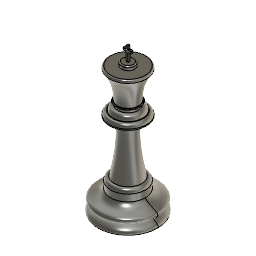
King (Autodesk Fusion 360 design; units mm, degrees)
part number: 2026-07-10-20-48-19-611
Autodesk Fusion 360 part; units mm, degrees
sketch "Pawn" plane through (0, 0, 0) normal (1, 0, 0) x (0, 1, 0)
  circle A0 through (0, 53, -10) (0, 61.6603, 5) (0, 44.3397, 5)
  line L0 (0, 43, 8.8) -> (0, 43, -8)
  line L1 (0, 40, -11) -> (0, 38.5991, -11)
  line L2 (0, 38.5991, -11) -> (0, 38.5991, 11.8)
  line L3 (0, 38.5991, 11.8) -> (0, 40, 11.8)
  arc A1 through (0, 43, 8.8) (0, 42.1213, 10.9213) (0, 40, 11.8)
  arc A2 through (0, 40, -11) (0, 42.1213, -10.1213) (0, 43, -8)
  arc A3 through (0, 13, 12) (0, 24.9602, 5.3081) (0, 38.5991, 3.9628)
  arc A4 through (0, 38.5991, -4.0372) (0, 24.9602, -5.3824) (0, 13, -12.0743)
  line L4 (0, 13, 14) -> (0, 13, -14)
  line L5 (0, 13, -14) -> (0, 9, -14)
  line L6 (0, 9, -14) -> (0, 9, 14)
  line L7 (0, 9, 14) -> (0, 13, 14)
  spline S0 degree 5 poles (0, 9, 14) (0, 8.9851, 14.1785) (0, 8.9515, 14.5305) (0, 8.8897, 15.0438) (0, 8.784, 15.698) (0, 8.6104, 16.4619) (0, 8.3911, 17.1666) (0, 8.1219, 17.8066) (0, 7.7992, 18.3771) (0, 7.4234, 18.8788) (0, 6.9978, 19.3158) (0, 6.6203, 19.6175) (0, 6.3176, 19.8184) (0, 6.1073, 19.9413) (0, 6, 20) knots 0 0 0 0 0 0 0.1 0.2 0.3 0.4 0.5 0.6 0.7 0.8 0.9 1 1 1 1 1 1
  spline S1 degree 5 poles (0, 9, -14) (0, 8.9851, -14.1785) (0, 8.9515, -14.5305) (0, 8.8897, -15.0438) (0, 8.784, -15.698) (0, 8.6104, -16.4619) (0, 8.3911, -17.1666) (0, 8.1219, -17.8066) (0, 7.7992, -18.3771) (0, 7.4234, -18.8788) (0, 6.9978, -19.3158) (0, 6.6203, -19.6175) (0, 6.3176, -19.8184) (0, 6.1073, -19.9413) (0, 6, -20) knots 0 0 0 0 0 0 0.1 0.2 0.3 0.4 0.5 0.6 0.7 0.8 0.9 1 1 1 1 1 1
  line L8 (0, 9.0732, -13.1224) -> (0, 8.9268, -14.8776)
  line L9 (0, 6.6579, -19.6402) -> (0, 5.3421, -20.3598)
  line L10 (0, 6, 20) -> (0, 6, 18)
  line L11 (0, 6, -20) -> (0, 6, -18)
  line L12 (0, 6, 18) -> (0, 6, -18)
  line L13 (0, 6, -18) -> (0, 4, -18)
  line L14 (0, 4, -18) -> (0, 4, 18)
  line L15 (0, 4, 18) -> (0, 6, 18)
  line L16 (0, 4, 19) -> (0, 4, -19)
  line L17 (0, 3, -20) -> (0, 0, -20)
  line L18 (0, 0, -20) -> (0, 0, 20)
  line L19 (0, 0, 20) -> (0, 3, 20)
  arc A5 through (0, 4, 19) (0, 3.7071, 19.7071) (0, 3, 20)
  arc A6 through (0, 3, -20) (0, 3.7071, -19.7071) (0, 4, -19)
  line L20 (0, 63) -> (0, 0)
  point P0 (0, 43)
  point P1 (0, 8)
  point P2 (0, 8)
  dimension "d1" = 3
  dimension "d2" = 3
  dimension "d3" = 1
  constraint coincident L20.end origin
sketch "Rook" plane through (0, 0, 0) normal (0, 1, 0) x (1, 0, 0)
  line L0 (-35, 0) -> (-21, 0)
  line L1 (-35, 0) -> (-21, 0)
  line L2 (-21, 0) -> (-21, -1.2451)
  line L3 (-21, -1.2451) -> (-35, -1.2451)
  line L4 (-35, -1.2451) -> (-35, 0)
  line L5 (-31.8127, -20) -> (-24.3127, -20)
  line L6 (-34.4949, -1.2451) -> (-21.5051, -1.2451)
  line L7 (-34.4949, -1.2451) -> (-21.5051, -1.2451)
  line L8 (-21.5051, -1.2451) -> (-21.5051, -1.8397)
  line L9 (-34.4949, -1.8397) -> (-34.4949, -1.2451)
  line L10 (-35, -1.8397) -> (-21.008, -1.8397)
  line L11 (-35, -1.8397) -> (-21, -1.8397)
  spline S0 degree 5 poles (-35, -1.8397) (-35.0093, -1.9913) (-35.017, -2.2834) (-34.9965, -2.6888) (-34.9076, -3.1639) (-34.711, -3.6512) (-34.4517, -4.0378) (-34.1537, -4.3344) (-33.8395, -4.559) (-33.5252, -4.7394) (-33.2213, -4.9103) (-32.9339, -5.1074) (-32.6663, -5.3627) (-32.42, -5.699) (-32.1955, -6.1278) (-31.9924, -6.6542) (-31.8468, -7.1538) (-31.7468, -7.572) (-31.6843, -7.8701) (-31.654, -8.024) knots 0 0 0 0 0 0 0.066667 0.133333 0.2 0.266667 0.333333 0.4 0.466667 0.533333 0.6 0.666667 0.733333 0.8 0.866667 0.933333 1 1 1 1 1 1
  line L12 (-34.916, -0.4639) -> (-35.084, -3.2156)
  spline S1 degree 5 poles (-21, -1.8397) (-20.9907, -1.9913) (-20.9832, -2.2831) (-21.0049, -2.6871) (-21.0964, -3.1589) (-21.2957, -3.6427) (-21.5551, -4.0292) (-21.8489, -4.3312) (-22.155, -4.566) (-22.4609, -4.757) (-22.7616, -4.9321) (-23.0554, -5.121) (-23.341, -5.3535) (-23.6134, -5.6567) (-23.863, -6.0541) (-24.0784, -6.5655) (-24.2144, -7.0781) (-24.2921, -7.5255) (-24.3325, -7.8522) (-24.3499, -8.0227) knots 0 0 0 0 0 0 0.066667 0.133333 0.2 0.266667 0.333333 0.4 0.466667 0.533333 0.6 0.666667 0.733333 0.8 0.866667 0.933333 1 1 1 1 1 1
  line L13 (-21.084, -0.4639) -> (-20.916, -3.2156)
  line L14 (-24.1985, -6.5384) -> (-24.5013, -9.5071)
  line L15 (-28, 0) -> (-28, -20)
  line L16 (-31.654, -8.024) -> (-24.3499, -8.0227)
  line L17 (-31.3947, -8.0234) -> (-24.6094, -8.0234)
  line L18 (-24.6094, -8.0234) -> (-24.6094, -8.4606)
  line L19 (-24.6094, -8.4606) -> (-31.3947, -8.4606)
  line L20 (-31.3947, -8.4606) -> (-31.3947, -8.0234)
  line L21 (-31.652, -8.4618) -> (-24.352, -8.4618)
  line L22 (-24.352, -8.4618) -> (-24.352, -9.381)
  line L23 (-24.352, -9.381) -> (-31.652, -9.381)
  line L24 (-31.652, -9.381) -> (-31.652, -8.4618)
  spline S2 degree 2 poles (-31.652, -9.381) (-32.2054, -9.8137) (-31.652, -10.1626) knots 0 0 0 0.114115 0.114115 0.114115 weights 1 3 1
  spline S3 degree 2 poles (-24.352, -9.381) (-23.7985, -9.8137) (-24.352, -10.1626) knots 0 0 0 0.114115 0.114115 0.114115 weights 1 3 1
  line L25 (-31.652, -10.1626) -> (-24.352, -10.1626)
  line L26 (-32.2054, -9.8137) -> (-23.7985, -9.8137)
  arc A0 (-30.5611, -15.016) -> (-31.652, -10.1626) centre (-41.3237, -14.8858) ccw
  arc A1 (-24.352, -10.1626) -> (-25.4428, -15.016) centre (-14.6802, -14.8858) ccw
  spline S4 degree 5 poles (-30.5611, -15.016) (-30.5652, -15.0447) (-30.5743, -15.1003) (-30.5907, -15.1783) (-30.6179, -15.2712) (-30.6611, -15.3691) (-30.7134, -15.4493) (-30.7748, -15.5129) (-30.8453, -15.5623) (-30.9245, -15.6011) (-31.0117, -15.6339) (-31.1052, -15.6655) (-31.2025, -15.7007) (-31.2991, -15.7436) (-31.389, -15.7968) (-31.4658, -15.8622) (-31.5244, -15.9401) (-31.5617, -16.0297) (-31.5789, -16.1292) (-31.5821, -16.235) (-31.5798, -16.3435) (-31.5821, -16.4503) (-31.5989, -16.5517) (-31.638, -16.6447) (-31.7016, -16.7241) (-31.7735, -16.7788) (-31.8387, -16.8145) (-31.8856, -16.8355) (-31.9075, -16.8445) knots 0 0 0 0 0 0 0.04 0.08 0.12 0.16 0.2 0.24 0.28 0.32 0.36 0.4 0.44 0.48 0.52 0.56 0.6 0.64 0.68 0.72 0.76 0.8 0.84 0.88 0.92 0.952038 0.952038 0.952038 0.952038 0.952038 0.952038
  spline S5 degree 5 poles (-30.5611, -15.016) (-30.5652, -15.0447) (-30.5743, -15.1003) (-30.5907, -15.1783) (-30.6179, -15.2712) (-30.6611, -15.3691) (-30.7134, -15.4493) (-30.7748, -15.5129) (-30.8453, -15.5623) (-30.9245, -15.6011) (-31.0117, -15.6339) (-31.1052, -15.6655) (-31.2025, -15.7007) (-31.2991, -15.7436) (-31.389, -15.7968) (-31.4658, -15.8622) (-31.5244, -15.9401) (-31.5617, -16.0297) (-31.5789, -16.1292) (-31.5821, -16.235) (-31.5798, -16.3435) (-31.5821, -16.4503) (-31.5989, -16.5517) (-31.638, -16.6447) (-31.7042, -16.7274) (-31.8003, -16.7988) (-31.902, -16.8464) (-31.9924, -16.8768) (-32.0588, -16.8948) (-32.0936, -16.9031) knots 0 0 0 0 0 0 0.04 0.08 0.12 0.16 0.2 0.24 0.28 0.32 0.36 0.4 0.44 0.48 0.52 0.56 0.6 0.64 0.68 0.72 0.76 0.8 0.84 0.88 0.92 0.96 1 1 1 1 1 1
  spline S6 degree 5 poles (-25.4441, -15.016) (-25.4399, -15.0447) (-25.4308, -15.1003) (-25.4143, -15.1783) (-25.387, -15.2712) (-25.3438, -15.3691) (-25.2914, -15.4492) (-25.2299, -15.5128) (-25.1594, -15.5621) (-25.0802, -15.6008) (-24.993, -15.6335) (-24.8994, -15.6651) (-24.8021, -15.7002) (-24.7055, -15.743) (-24.6155, -15.7962) (-24.5386, -15.8615) (-24.4801, -15.9393) (-24.4427, -16.029) (-24.4253, -16.1284) (-24.4221, -16.2343) (-24.4244, -16.3427) (-24.4219, -16.4495) (-24.4051, -16.5509) (-24.3659, -16.6439) (-24.3023, -16.7232) (-24.2303, -16.7778) (-24.1652, -16.8135) (-24.1183, -16.8344) (-24.0964, -16.8434) knots 0 0 0 0 0 0 0.04 0.08 0.12 0.16 0.2 0.24 0.28 0.32 0.36 0.4 0.44 0.48 0.52 0.56 0.6 0.64 0.68 0.72 0.76 0.8 0.84 0.88 0.92 0.952001 0.952001 0.952001 0.952001 0.952001 0.952001
  line L27 (-25.4978, -14.6424) -> (-25.3904, -15.3895)
  line L28 (-23.9101, -17.121) -> (-23.9101, -18.0867)
  line L29 (-23.9101, -18.0867) -> (-32.0936, -18.0867)
  line L30 (-32.0936, -18.0867) -> (-32.0936, -17.122)
  arc A2 (-31.9075, -16.8445) -> (-32.0936, -17.122) centre (-31.7936, -17.122) ccw
  arc A3 (-23.9101, -17.121) -> (-24.0964, -16.8434) centre (-24.2101, -17.121) ccw
  line L31 (-24.1115, -18.0867) -> (-24.1115, -18.2621)
  line L32 (-24.1115, -18.2621) -> (-31.8922, -18.2621)
  line L33 (-31.8922, -18.2621) -> (-31.8922, -18.0867)
  line L34 (-32.0938, -18.2621) -> (-23.9098, -18.2621)
  line L35 (-32.0938, -18.2621) -> (-23.9101, -18.2621)
  line L36 (-23.9101, -18.2621) -> (-23.9101, -19.9954)
  line L37 (-23.9101, -19.9954) -> (-32.0938, -19.9954)
  line L38 (-32.0938, -19.9954) -> (-32.0938, -18.2621)
  point P0 (-28, -1.2451)
  point P1 (-28.004, -1.8397)
  point P2 (-34.0723, -4.3805)
  point P3 (-32.7952, -5.2511)
  point P4 (-21.9277, -4.3805)
  point P5 (-23.2048, -5.2511)
  point P6 (-28.002, -8.0234)
  point P7 (-27.9788, -8.4606)
  point P8 (-30.7809, -15.5126)
  point P9 (-31.1893, -15.6974)
  point P10 (-31.5491, -16.0085)
  point P11 (-31.5977, -16.5239)
  point P12 (-31.5491, -16.0085)
  point P13 (-31.5977, -16.5239)
  point P14 (-31.1893, -15.6974)
  point P15 (-30.7809, -15.5126)
  point P16 (-25.2239, -15.5125)
  point P17 (-24.8153, -15.6969)
  point P18 (-24.4553, -16.0078)
  point P19 (-24.4063, -16.5231)
  point P20 (-28.0018, -18.0867)
  point P21 (-28.0018, -18.2621)
  dimension "d23" = 14
  dimension "d27" = 0.3
  dimension "d28" = 0.3
  dimension "d29" = 8.184
  constraint horizontal L0
  constraint horizontal L1
  constraint vertical L2
  constraint horizontal L3
  constraint vertical L4
  constraint horizontal L5
  constraint midpoint L6 P0
  constraint coincident L3 P0
  constraint coincident L3 L6.end
  constraint horizontal L7
  constraint vertical L8
  constraint vertical L9
  constraint midpoint L10 P1
  constraint perpendicular L8 L10
  constraint horizontal L11
  constraint midpoint L10.start L12
  constraint midpoint L1 L15.start
  constraint coincident L5 L15.end
  constraint perpendicular L5 L15
  constraint midpoint L17 P6
  constraint coincident L16 P6
  constraint perpendicular L15 L17
  constraint vertical L18
  constraint horizontal L19
  constraint vertical L20
  constraint coincident L19 P7
  constraint horizontal L21
  constraint vertical L22
  constraint horizontal L23
  constraint vertical L24
  constraint parallel L23 L25
  constraint perpendicular L15 L26
  constraint vertical L28
  constraint horizontal L29
  constraint vertical L30
  constraint tangent L30 A2
  constraint tangent S4 A2
  constraint tangent S6 A3
  constraint tangent L28 A3
  constraint coincident L29 P20
  constraint vertical L31
  constraint horizontal L32
  constraint vertical L33
  constraint midpoint L34 P21
  constraint coincident L32 P21
  constraint perpendicular L15 L34
  constraint horizontal L35
  constraint vertical L36
  constraint horizontal L37
  constraint vertical L38
  measures "d23" distance of L0.start L0.end
  measures "d27" radius of A2
  measures "d28" radius of A3
  measures "d29" distance of L34.start L34.end
sketch "Rook Dip" plane through (0, 0, 19.9954) normal (0, 0, 1) x (-1, 0, 0)
  circle A0 centre (28, 0) radius 4.0938
  circle A1 centre (28, 0) radius 3.437
  constraint concentric A0 A1
sketch "Rook Notches Direction 1" plane through (0, 0, 0) normal (0, 1, 0) x (1, 0, 0)
  line L0 (-32.0944, -20.0834) -> (-23.9073, -20.0834)
  line L1 (-28.0008, -20.0834) -> (-28.0008, -18.7054)
  line L2 (-28.9156, -20.0834) -> (-27.0861, -20.0834)
  line L3 (-28.6168, -18.7054) -> (-27.3849, -18.7054)
  line L4 (-28.9156, -20.0834) -> (-28.6168, -18.7054)
  line L5 (-27.3849, -18.7054) -> (-27.0861, -20.0834)
  point P0 (-28.0008, -18.7054)
  constraint horizontal L0
  constraint midpoint L0 L1.start
  constraint perpendicular L0 L1
  constraint midpoint L1.start L2
  constraint coincident L0 L2.end
  constraint midpoint L3 P0
  constraint coincident L1 P0
  constraint perpendicular L1 L3
  constraint coincident P0 L1.end
sketch "Rook Notches Direction 2" plane through (0, 0, 0) normal (1, 0, 0) x (0, 1, 0)
  line L0 (-28.9156, -20.0834) -> (-28.6168, -18.7054)
  line L1 (-28.9156, -20.0834) -> (-27.0861, -20.0834)
  line L2 (-28.6168, -18.7054) -> (-27.3849, -18.7054)
  line L3 (-27.3849, -18.7054) -> (-27.0861, -20.0834)
  line L4 (-28.9156, -20.0834) -> (-28.6168, -18.7054)
  line L5 (-28.9156, -20.0834) -> (-27.0861, -20.0834)
  line L6 (-28.6168, -18.7054) -> (-27.3849, -18.7054)
  line L7 (-27.3849, -18.7054) -> (-27.0861, -20.0834)
  line L8 (0.616, 18.7045, -28.1694) -> (-0.616, 18.7045, -28.1694)
  line L9 (0.915, 20.0825, -28.1694) -> (-0.915, 20.0825, -28.1694)
  line L10 (0.915, 20.0825, -28.1694) -> (0.616, 18.7045, -28.1694)
  line L11 (-0.616, 18.7045, -28.1694) -> (-0.915, 20.0825, -28.1694)
  point P0 (0, 20)
  dimension "d42" = 1.232
  dimension "d43" = 1.83
sketch "Queen" plane through (0, 0, 0) normal (0, 1, 0) x (1, 0, 0)
  line L0 (-7.5, 0) -> (7.5, 0)
  line L1 (0, 0) -> (0, -30)
  line L2 (-7.5, 0) -> (7.5, 0)
  line L3 (-4.5355, -1.5) -> (5.25, -1.5)
  arc A0 (-7.5, 0) -> (-5.25, -1.5) centre (-5.25, 0.9375) ccw
  arc A1 (5.25, -1.5) -> (7.5, 0) centre (5.25, 0.9375) ccw
  line L4 (-5.25, -1.5) -> (4.5355, -1.5)
  arc A2 (-4.5355, -1.5) -> (-5.25, -2.2145) centre (-4.5355, -2.2145) ccw
  arc A3 (5.25, -2.2145) -> (4.5355, -1.5) centre (4.5355, -2.2145) ccw
  line L5 (0, -1.5) -> (0, -7.5)
  line L6 (-4, -7.5) -> (4, -7.5)
  arc A4 (-4, -7.5) -> (-5.25, -2.2145) centre (-13.401, -6.9327) ccw
  arc A5 (5.25, -2.2145) -> (4, -7.5) centre (13.401, -6.9327) ccw
  line L7 (-3.75, -7.5) -> (3.75, -7.5)
  line L8 (-2.5, -22.5) -> (2.5, -22.5)
  arc A6 (3.75, -7.5) -> (2.5, -22.5) centre (72.7579, -20.8027) ccw
  arc A7 (-2.5, -22.5) -> (-3.75, -7.5) centre (-72.9542, -20.8191) ccw
  line L9 (-5, -22.5) -> (5, -22.5)
  line L10 (-5, -22.5) -> (5, -22.5)
  line L11 (5, -22.5) -> (5, -22.5353)
  line L12 (3.9353, -23.6) -> (-3.9353, -23.6)
  line L13 (-5, -22.5353) -> (-5, -22.5)
  arc A8 (-5, -22.5353) -> (-3.9353, -23.6) centre (-3.9353, -22.5353) ccw
  arc A9 (3.9353, -23.6) -> (5, -22.5353) centre (3.9353, -22.5353) ccw
  line L14 (-3.9353, -23.6) -> (3.9353, -23.6)
  line L15 (-3.9353, -23.6) -> (3.9353, -23.6)
  line L16 (3.9353, -23.6) -> (3.9353, -23.8711)
  line L17 (-3.9353, -23.8711) -> (-3.9353, -23.6)
  arc A10 (-3.9353, -23.8711) -> (-3.1064, -24.7) centre (-3.1064, -23.8711) ccw
  arc A11 (3.1064, -24.7) -> (3.9353, -23.8711) centre (3.1064, -23.8711) ccw
  line L18 (-3.1064, -24.7) -> (3.1064, -24.7)
  line L19 (-2.5, -24.7) -> (2.5, -24.7)
  line L20 (-2.5, -24.7) -> (2.5, -24.7)
  line L21 (2.5, -24.7) -> (2.5, -25)
  line L22 (2.5, -25) -> (-2.5, -25)
  line L23 (-2.5, -25) -> (-2.5, -24.7)
  line L24 (-2.6615, -25) -> (2.6615, -25)
  line L25 (2.8, -25.1385) -> (2.8, -25.1615)
  line L26 (2.6615, -25.3) -> (-2.6615, -25.3)
  line L27 (-2.8, -25.1615) -> (-2.8, -25.1385)
  arc A12 (-2.6615, -25) -> (-2.8, -25.1385) centre (-2.6615, -25.1385) ccw
  arc A13 (-2.8, -25.1615) -> (-2.6615, -25.3) centre (-2.6615, -25.1615) ccw
  arc A14 (2.6615, -25.3) -> (2.8, -25.1615) centre (2.6615, -25.1615) ccw
  arc A15 (2.8, -25.1385) -> (2.6615, -25) centre (2.6615, -25.1385) ccw
  line L28 (-2.5, -25.3) -> (2.5, -25.3)
  line L29 (0, -30) -> (0, -32.5)
  line L30 (-4.5, -32.5) -> (4.5, -32.5)
  line L31 (-4.5, -32.5) -> (-2.5, -25.3)
  line L32 (4.5, -32.5) -> (2.5, -25.3)
  point P0 (0, -1.5)
  point P1 (0, -22.5)
  point P2 (0, -22.5)
  point P3 (-5, -23.6)
  point P4 (0, -23.6)
  point P5 (-3.9353, -24.7)
  point P6 (0, -24.7)
  point P7 (0, -24.7)
  point P8 (-2.8, -25)
  point P9 (2.8, -25)
  point P10 (0, -25)
  point P11 (-2.8, -25.3)
  point P12 (0, -25.3)
  dimension "d48" = 15
  dimension "d51" = 10.5
  dimension "d53" = 0.7145
  dimension "d55" = 8
  dimension "d56" = 7.5
  dimension "d57" = 5
  dimension "d58" = 10
  dimension "d59" = 1.1
  dimension "d60" = 1.0647
  dimension "d61" = 1.1
  dimension "d62" = 0.8289
  dimension "d63" = 5
  dimension "d64" = 5.6
  dimension "d65" = 0.3
  dimension "d66" = 0.1385
  dimension "d67" = 5
  dimension "d68" = 9
  constraint midpoint L0 L1.start
  constraint coincident L1.start origin
  constraint horizontal L0
  constraint perpendicular L0 L1
  constraint horizontal L2
  constraint coincident L1 P0
  constraint perpendicular L1 L3
  constraint tangent L3 A0
  constraint tangent L3 A1
  constraint horizontal L4
  constraint coincident L3 P0
  constraint coincident A0.end L3
  constraint tangent L3 A2
  constraint tangent L4 A3
  constraint equal A2 A3
  constraint coincident P0 L5.start
  constraint coincident L1 L5.end
  constraint midpoint L5.end L6
  constraint perpendicular L1 L6
  constraint midpoint L5.end L7
  constraint perpendicular L1 L7
  constraint midpoint L8 P2
  constraint coincident L1 P2
  constraint perpendicular L1 L8
  constraint midpoint L9 P2
  constraint coincident P2 P1
  constraint perpendicular L1 L9
  constraint horizontal L10
  constraint vertical L11
  constraint horizontal L12
  constraint vertical L13
  constraint coincident P3 L12
  constraint coincident P3 L13
  constraint tangent L12 A8
  constraint tangent L13 A8
  constraint tangent L11 A9
  constraint tangent L12 A9
  constraint equal A8 A9
  constraint midpoint L14 P4
  constraint coincident L12 P4
  constraint horizontal L15
  constraint vertical L16
  constraint vertical L17
  constraint coincident P5 L17
  constraint tangent L17 A10
  constraint tangent L16 A11
  constraint equal A10 A11
  constraint tangent A11 L18
  constraint midpoint L19 P7
  constraint coincident P7 P6
  constraint perpendicular L1 L19
  constraint horizontal L20
  constraint vertical L21
  constraint horizontal L22
  constraint vertical L23
  constraint coincident L22 P10
  constraint perpendicular L21 L24
  constraint vertical L25
  constraint horizontal L26
  constraint vertical L27
  constraint coincident L24 P10
  constraint coincident P8 L24
  constraint coincident P8 L27
  constraint tangent L24 A12
  constraint tangent L27 A12
  constraint coincident P11 L26
  constraint coincident P11 L27
  constraint tangent L26 A13
  constraint tangent L27 A13
  constraint equal A12 A13
  constraint tangent L25 A14
  constraint tangent L26 A14
  constraint equal A12 A14
  constraint coincident P9 L24
  constraint tangent L25 A15
  constraint tangent L24 A15
  constraint equal A12 A15
  constraint midpoint L28 P12
  constraint coincident L26 P12
  constraint parallel L26 L28
  constraint parallel L1 L29
  constraint midpoint L29.end L30
  constraint perpendicular L29 L30
  measures "d48" distance of L0.start L0.end
  measures "d51" distance of A0.end L3.end
  measures "d53" radius of A2
  measures "d55" distance of L6.start L6.end
  measures "d56" distance of L7.start L7.end
  measures "d57" distance of L8.start L8.end
  measures "d58" distance of L9.start L9.end
  measures "d59" distance of L9.start P3
  measures "d60" radius of A8
  measures "d61" distance of L12.end P5
  measures "d62" radius of A10
  measures "d63" distance of L19.start L19.end
  measures "d64" distance of P8 P9
  measures "d65" distance of P8 P11
  measures "d66" radius of A12
  measures "d67" distance of L28.start L28.end
  measures "d68" distance of L30.start L30.end
sketch "Queen Dip" plane through (0, 0, 0) normal (0, 1, 0) x (1, 0, 0)
  line L0 (-3.5, -32.5) -> (3.5, -32.5)
  line L1 (-1.5, -25.3) -> (1.5, -25.3)
  line L2 (-3.5, -32.5) -> (-1.5, -25.3)
  line L3 (1.5, -25.3) -> (3.5, -32.5)
  line L4 (0, -32.5) -> (0, -25.3)
  circle A0 centre (0, -32.5) radius 1.8
  point P0 (0, -32.5)
  point P1 (0, -25.3)
  dimension "d70" = 7
  dimension "d71" = 3
  constraint midpoint L0 P0
  constraint horizontal L0
  constraint midpoint L1 P1
  constraint horizontal L1
  constraint coincident P0 L4.start
  constraint coincident P1 L4.end
  constraint perpendicular L1 L4
  measures "d70" distance of L0.start L0.end
  measures "d71" distance of L1.start L1.end
ref_plane "WorkPlane1" through (0, -4.5, 28.9) normal (0, 1, 0) x (0, 0, 1)
sketch "Queen Head" plane through (0, -4.5, 0) normal (0, 1, 0) x (1, 0, 0)
  circle A0 centre (0, -32.5) radius 1.8
  dimension "d75" = 3.6
  measures "d75" diameter of A0
ref_plane "WorkPlane2" through (0, 0, 28.9008) normal (0, 1, 0) x (0, 0, 1)
sketch "Queen Details" plane through (0, 0, 0) normal (0, 1, 0) x (1, 0, 0)
  line L0 (-2.6192, -32.5) -> (2.6192, -32.5)
  line L1 (0, -32.5) -> (0, -30.5)
  line L2 (-3, -30.5) -> (3, -30.5)
  arc A0 (-3, -30.5) -> (3, -30.5) centre (0, -30.5) ccw
  line L3 (0, -32.5) -> (0, -35)
  line L4 (-0.45, -33.4) -> (0.45, -33.4)
  line L5 (-0.65, -35) -> (-0.45, -33.4)
  line L6 (0.45, -33.4) -> (0.65, -35)
  line L7 (-0.65, -35) -> (-0.55, -35)
  line L8 (0.65, -35) -> (0.55, -35)
  arc A1 (0.55, -35) -> (-0.55, -35) centre (0, -35) ccw
  point P0 (0, -32.5)
  point P1 (0, -33.4)
  dimension "d82" = 2
  dimension "d83" = 6
  dimension "d84" = 2.5
  dimension "d85" = 1.3
  dimension "d86" = 0.9
  constraint midpoint L0 P0
  constraint horizontal L0
  constraint coincident P0 L1.start
  constraint perpendicular L0 L1
  constraint midpoint L1.end L2
  constraint perpendicular L1 L2
  constraint coincident L1.end A0.centre
  constraint perpendicular L0 L3
  constraint midpoint L4 P1
  constraint coincident L3 P1
  constraint perpendicular L3 L4
  constraint horizontal L7
  constraint horizontal L8
  constraint coincident L3.end A1.centre
  measures "d82" distance of P0 L1.end
  measures "d83" distance of L2.start L2.end
  measures "d84" distance of P0 L3.end
  measures "d85" distance of L5.start L6.end
  measures "d86" distance of L4.start L4.end
ref_plane "WorkPlane3" through (0, -0.65, 34.2324) normal (0, 1, 0) x (0, 0, 1)
sketch "Bishop" plane through (0, 0, 0) normal (0, 1, 0) x (1, 0, 0)
  line L0 (-7, 0) -> (7, 0)
  line L1 (-15, -27.5) -> (15, -27.5)
  line L2 (-7, 0) -> (7, 0)
  line L3 (7, 0) -> (7, -1)
  line L4 (7, -1) -> (-7, -1)
  line L5 (-7, -1) -> (-7, 0)
  line L6 (0, 0) -> (0, -27.5)
  line L7 (-6.5, -1) -> (6.5, -1)
  line L8 (-6.5, -1) -> (6.5, -1)
  line L9 (6.5, -1) -> (6.5, -1.5)
  line L10 (6.5, -1.5) -> (-6.5, -1.5)
  line L11 (-6.5, -1.5) -> (-6.5, -1)
  line L12 (-7, -1.5) -> (7, -1.5)
  line L13 (-7, -1.5) -> (7, -1.5)
  line L14 (0, -1.5) -> (0, -6.5)
  line L15 (0, -1.5) -> (0, -6.5)
  spline S0 degree 5 poles (-7, -1.5) (-7.0246, -1.5806) (-7.0703, -1.7382) (-7.1286, -1.9634) (-7.1789, -2.2302) (-7.1668, -2.472) (-7.0538, -2.6012) (-6.847, -2.6833) (-6.5825, -2.832) (-6.2651, -3.0287) (-5.9052, -3.2414) (-5.5169, -3.4296) (-5.152, -3.6359) (-4.8656, -3.9317) (-4.6833, -4.345) (-4.6202, -4.8953) (-4.6685, -5.4488) (-4.7603, -5.9277) (-4.8459, -6.2752) (-4.8948, -6.4559) knots 0 0 0 0 0 0 0.066667 0.133333 0.2 0.266667 0.333333 0.4 0.466667 0.533333 0.6 0.666667 0.733333 0.8 0.866667 0.933333 1 1 1 1 1 1
  line L16 (-7.3838, -2.3732) -> (-6.6162, -2.8469)
  line L17 (-6.6598, -0.3839) -> (-7.3402, -2.6161)
  spline S1 degree 5 poles (-7, -1.5) (-7.0254, -1.5833) (-7.0723, -1.7439) (-7.1308, -1.9666) (-7.1799, -2.2235) (-7.1642, -2.4655) (-7.0415, -2.6214) (-6.7895, -2.7071) (-6.4171, -2.7601) (-5.9647, -2.816) (-5.4873, -2.9121) (-5.0444, -3.0809) (-4.6868, -3.3479) (-4.4459, -3.727) (-4.3386, -4.2246) (-4.3718, -4.8417) (-4.5114, -5.4297) (-4.6789, -5.9227) (-4.8182, -6.2743) (-4.8948, -6.4559) knots 0 0 0 0 0 0 0.066667 0.133333 0.2 0.266667 0.333333 0.4 0.466667 0.533333 0.6 0.666667 0.733333 0.8 0.866667 0.933333 1 1 1 1 1 1
  line L18 (-6.6598, -0.3839) -> (-7.3402, -2.6161)
  line L19 (-7.3838, -2.3732) -> (-6.6162, -2.8469)
  line L20 (-4.8948, -6.4559) -> (4.8952, -6.4559)
  line L21 (0, -6.5) -> (0, -7.5)
  line L22 (-4.8948, -6.4559) -> (0, -7.5)
  line L23 (4.8952, -6.4559) -> (0, -7.5)
  line L24 (-3.3979, -6.7753) -> (3.3979, -6.7753)
  line L25 (0, -6.5) -> (0, -14)
  line L26 (-2.0655, -14) -> (2.0655, -14)
  arc A0 (-2.4301, -13.5777) -> (-3.3979, -6.7753) centre (-14.407, -11.8116) ccw
  arc A1 (3.3979, -6.7753) -> (2.4301, -13.5777) centre (14.407, -11.8116) ccw
  line L27 (-6.1022, -3.1214) -> (-4.965, -3.7357)
  arc A2 (-2.4301, -13.5777) -> (-2.0655, -14) centre (-2.0655, -13.6314) ccw
  arc A3 (2.0655, -14) -> (2.4301, -13.5777) centre (2.0655, -13.6314) ccw
  line L28 (-4, -14) -> (4, -14)
  line L29 (-4, -14) -> (4, -14)
  line L30 (4, -14) -> (4, -14.1154)
  line L31 (3.4154, -14.7) -> (-3.4154, -14.7)
  line L32 (-4, -14.1154) -> (-4, -14)
  arc A4 (-4, -14.1154) -> (-3.4154, -14.7) centre (-3.4154, -14.1154) ccw
  arc A5 (3.4154, -14.7) -> (4, -14.1154) centre (3.4154, -14.1154) ccw
  line L33 (-3, -14.7) -> (3, -14.7)
  line L34 (-3, -14.7) -> (3, -14.7)
  line L35 (3, -14.7) -> (3, -14.6535)
  line L36 (2.2535, -15.4) -> (-2.2535, -15.4)
  line L37 (-3, -14.6535) -> (-3, -14.7)
  arc A6 (-3, -14.6535) -> (-2.2535, -15.4) centre (-2.2535, -14.6535) ccw
  arc A7 (2.2535, -15.4) -> (3, -14.6535) centre (2.2535, -14.6535) ccw
  line L38 (-2.2978, -15.4) -> (2.2978, -15.4)
  line L39 (-2.2978, -15.4) -> (2.2978, -15.4)
  line L40 (2.2978, -15.4) -> (2.2978, -15.6)
  line L41 (2.2978, -15.6) -> (-2.1206, -15.6)
  line L42 (-2.2978, -15.6) -> (-2.2978, -15.4)
  line L43 (-2.4, -15.6) -> (2.4, -15.6)
  line L44 (-2.4, -15.6) -> (2.1206, -15.6)
  line L45 (2.4, -15.8794) -> (2.4, -15.9206)
  line L46 (2.1206, -16.2) -> (-2.1206, -16.2)
  line L47 (-2.4, -15.9206) -> (-2.4, -15.8794)
  arc A8 (-2.4, -15.9206) -> (-2.1206, -16.2) centre (-2.1206, -15.9206) ccw
  arc A9 (-2.1206, -15.6) -> (-2.4, -15.8794) centre (-2.1206, -15.8794) ccw
  arc A10 (2.4, -15.8794) -> (2.1206, -15.6) centre (2.1206, -15.8794) ccw
  arc A11 (2.1206, -16.2) -> (2.4, -15.9206) centre (2.1206, -15.9206) ccw
  line L48 (-2.1206, -16.2) -> (2.1206, -16.2)
  line L49 (0, -27.5) -> (0, -25.5)
  line L50 (0, -25.5) -> (0, -16.2)
  line L51 (-4, -20.85) -> (4, -20.85)
  line L52 (-2.1206, -16.2) -> (-4, -20.85)
  line L53 (2.1206, -16.2) -> (4, -20.85)
  line L54 (-1, -25.5) -> (1, -25.5)
  line L55 (-4, -20.85) -> (-1, -25.5)
  line L56 (1, -25.5) -> (4, -20.85)
  line L57 (-1, -25.5) -> (1, -25.5)
  line L58 (1, -25.5) -> (1, -25.7)
  line L59 (-1, -25.7) -> (-1, -25.5)
  line L60 (1.5, -26.1153) -> (1.5, -26.3847)
  line L61 (1.0847, -26.8) -> (-1.0847, -26.8)
  line L62 (-1.5, -26.3847) -> (-1.5, -26.1153)
  arc A12 (-1.0847, -25.7) -> (-1.5, -26.1153) centre (-1.0847, -26.1153) ccw
  arc A13 (1.5, -26.1153) -> (1.0847, -25.7) centre (1.0847, -26.1153) ccw
  arc A14 (1.0847, -26.8) -> (1.5, -26.3847) centre (1.0847, -26.3847) ccw
  arc A15 (-1.5, -26.3847) -> (-1.0847, -26.8) centre (-1.0847, -26.3847) ccw
  line L63 (-1, -25.7) -> (1, -25.7)
  line L64 (1.0847, -25.7) -> (1, -25.7)
  point P0 (0, -27.5)
  point P1 (0, -1)
  point P2 (0, -1.5)
  point P3 (-7, -2.6101)
  point P4 (-5.5336, -3.4285)
  point P5 (-7, -2.6101)
  point P6 (-5.0803, -3.0972)
  point P7 (0, -6.7753)
  point P8 (-2.5, -14)
  point P9 (2.5, -14)
  point P10 (-4, -14.7)
  point P11 (0, -14.7)
  point P12 (-3, -15.4)
  point P13 (0, -15.4)
  point P14 (0, -15.6)
  point P15 (-2.4, -16.2)
  point P16 (0, -16.2)
  point P17 (0, -20.85)
  point P18 (0, -25.7)
  point P19 (-1.5, -26.8)
  dimension "d101" = 14
  dimension "d102" = 5
  dimension "d104" = 7.5
  dimension "d105" = 5
  dimension "d106" = 0.3686
  dimension "d107" = 8
  dimension "d108" = 0.7
  dimension "d109" = 0.5846
  dimension "d110" = 6
  dimension "d111" = 0.7
  dimension "d112" = 0.7465
  dimension "d113" = 0.2
  dimension "d114" = 4.8
  dimension "d115" = 0.6
  dimension "d116" = 0.2794
  dimension "d117" = 2
  dimension "d118" = 9.3
  dimension "d119" = 8
  dimension "d120" = 2
  dimension "d121" = 0.2
  dimension "d124" = 0.4153
  constraint midpoint L0 L6.start
  constraint coincident L6.start origin
  constraint horizontal L0
  constraint midpoint L1 P0
  constraint horizontal L1
  constraint horizontal L2
  constraint vertical L3
  constraint horizontal L4
  constraint vertical L5
  constraint coincident P0 L6.end
  constraint perpendicular L1 L6
  constraint midpoint L7 P1
  constraint coincident L4 P1
  constraint coincident L4 L7.end
  constraint horizontal L8
  constraint vertical L9
  constraint horizontal L10
  constraint vertical L11
  constraint midpoint L12 P2
  constraint coincident L10 P2
  constraint perpendicular L6 L12
  constraint horizontal L13
  constraint coincident P2 L14.start
  constraint coincident L6 L14.end
  constraint midpoint P5 L16
  constraint midpoint L12.start L17
  constraint midpoint P5 L19
  constraint midpoint L12.start L18
  constraint horizontal L20
  constraint coincident L6 L21.end
  constraint midpoint L24 P7
  constraint coincident L21 P7
  constraint coincident L23 L24.end
  constraint perpendicular L21 L24
  constraint perpendicular L24 L25
  constraint perpendicular L6 L26
  constraint midpoint P4 L27
  constraint coincident L25.end L26
  constraint coincident P8 L26
  constraint coincident P8 A0
  constraint tangent L26 A2
  constraint tangent A0 A2
  constraint tangent A1 A3
  constraint tangent L26 A3
  constraint equal A2 A3
  constraint midpoint L25.end L28
  constraint perpendicular L25 L28
  constraint horizontal L29
  constraint vertical L30
  constraint horizontal L31
  constraint vertical L32
  constraint coincident P10 L31
  constraint coincident P10 L32
  constraint tangent L31 A4
  constraint tangent L32 A4
  constraint tangent L30 A5
  constraint tangent L31 A5
  constraint equal A4 A5
  constraint midpoint L33 P11
  constraint coincident L31 P11
  constraint perpendicular L6 L33
  constraint horizontal L34
  constraint vertical L35
  constraint horizontal L36
  constraint vertical L37
  constraint coincident P12 L36
  constraint coincident P12 L37
  constraint tangent L36 A6
  constraint tangent L37 A6
  constraint tangent L35 A7
  constraint tangent L36 A7
  constraint equal A6 A7
  constraint midpoint L38 P13
  constraint coincident L36 P13
  constraint perpendicular L6 L38
  constraint horizontal L39
  constraint vertical L40
  constraint horizontal L41
  constraint vertical L42
  constraint midpoint L43 P14
  constraint coincident L41 P14
  constraint perpendicular L40 L43
  constraint horizontal L44
  constraint vertical L45
  constraint horizontal L46
  constraint vertical L47
  constraint coincident P15 L46
  constraint coincident P15 L47
  constraint tangent L46 A8
  constraint tangent L47 A8
  constraint coincident L43.start L47
  constraint coincident L42.start L41
  constraint tangent L47 A9
  constraint tangent L41 A9
  constraint equal A8 A9
  constraint tangent L44 A10
  constraint tangent L45 A10
  constraint equal A8 A10
  constraint tangent L45 A11
  constraint tangent L46 A11
  constraint equal A8 A11
  constraint midpoint L48 P16
  constraint coincident L46 P16
  constraint perpendicular L1 L49
  constraint perpendicular L46 L50
  constraint midpoint L51 P17
  constraint coincident L50 P17
  constraint perpendicular L50 L51
  constraint midpoint L49.end L54
  constraint perpendicular L50 L54
  constraint horizontal L57
  constraint vertical L58
  constraint vertical L59
  constraint vertical L60
  constraint horizontal L61
  constraint vertical L62
  constraint tangent L62 A12
  constraint tangent L60 A13
  constraint equal A12 A13
  constraint tangent L60 A14
  constraint tangent L61 A14
  constraint equal A12 A14
  constraint coincident P19 L61
  constraint coincident P19 L62
  constraint tangent L61 A15
  constraint tangent L62 A15
  constraint equal A12 A15
  constraint perpendicular L58 L63
  constraint tangent A13 L64
  measures "d101" distance of L0.start L0.end
  measures "d102" distance of P2 L14.end
  measures "d104" distance of L14.end L25.end
  measures "d105" distance of P8 P9
  measures "d106" radius of A2
  measures "d107" distance of L28.start L28.end
  measures "d108" distance of L28.start P10
  measures "d109" radius of A4
  measures "d110" distance of L33.start L33.end
  measures "d111" distance of L33.start P12
  measures "d112" radius of A6
  measures "d113" distance of L38.start L42.start
  measures "d114" distance of L43.start L43.end
  measures "d115" distance of L43.start P15
  measures "d116" radius of A8
  measures "d117" distance of P0 L49.end
  measures "d118" distance of L49.end P16
  measures "d119" distance of L51.start L51.end
  measures "d120" distance of L54.start L54.end
  measures "d121" distance of L54.start L59.start
  measures "d124" radius of A12
sketch "King" plane through (0, 0, 0) normal (0, 1, 0) x (1, 0, 0)
  line L0 (-8, 0) -> (8, 0)
  line L1 (0, 0) -> (0, -37)
  line L2 (-5.5, -34.0205) -> (5.5, -34.0205)
  line L3 (-6, -2) -> (6, -2)
  spline S0 degree 5 poles (-8, 0) (-8.0444, -0.05) (-8.1187, -0.1535) (-8.1868, -0.3192) (-8.1848, -0.5626) (-7.9522, -0.9222) (-7.4658, -1.2823) (-6.8474, -1.6136) (-6.3043, -1.8659) (-6, -2) knots 0 0 0 0 0 0 0.2 0.4 0.6 0.8 1 1 1 1 1 1
  line L4 (-6.7505, -1.6693) -> (-5.2495, -2.3307)
  spline S1 degree 5 poles (8, 0) (8.0444, -0.05) (8.1187, -0.1535) (8.1868, -0.3192) (8.1848, -0.5626) (7.9522, -0.9222) (7.4658, -1.2823) (6.8474, -1.6136) (6.3043, -1.8659) (6, -2) knots 0 0 0 0 0 0 0.2 0.4 0.6 0.8 1 1 1 1 1 1
  line L5 (7.923, 0.0867) -> (8.077, -0.0867)
  line L6 (6.7505, -1.6693) -> (5.2495, -2.3307)
  spline S2 degree 5 poles (-6, -2) (-6.078, -1.9867) (-6.2314, -1.9655) (-6.4537, -1.9499) (-6.7346, -1.9615) (-7.0587, -2.0299) (-7.3527, -2.1501) (-7.6109, -2.3172) (-7.8246, -2.5217) (-7.9806, -2.7482) (-8.0652, -2.9789) (-8.0668, -3.1977) (-7.9797, -3.3933) (-7.8081, -3.5643) (-7.5641, -3.7169) (-7.2642, -3.8623) (-6.9262, -4.0132) (-6.566, -4.1811) (-6.1945, -4.3734) (-5.8191, -4.5948) (-5.4438, -4.8476) (-5.1455, -5.0756) (-4.9232, -5.2611) (-4.7756, -5.3912) (-4.7019, -5.4579) knots 0 0 0 0 0 0 0.05 0.1 0.15 0.2 0.25 0.3 0.35 0.4 0.45 0.5 0.55 0.6 0.65 0.7 0.75 0.8 0.85 0.9 0.95 1 1 1 1 1 1
  spline S3 degree 5 poles (6, -2) (6.0773, -1.9865) (6.2296, -1.9649) (6.4513, -1.9493) (6.7329, -1.9616) (7.0589, -2.0312) (7.3544, -2.152) (7.6124, -2.3183) (7.824, -2.5208) (7.9774, -2.7453) (8.0608, -2.9758) (8.0645, -3.1974) (7.9828, -3.3989) (7.8175, -3.5765) (7.5769, -3.733) (7.2734, -3.8757) (6.9223, -4.0154) (6.54, -4.164) (6.1426, -4.334) (5.7453, -4.5372) (5.3612, -4.7844) (5.0731, -5.0242) (4.8709, -5.2305) (4.7427, -5.3801) (4.6802, -5.4579) knots 0 0 0 0 0 0 0.05 0.1 0.15 0.2 0.25 0.3 0.35 0.4 0.45 0.5 0.55 0.6 0.65 0.7 0.75 0.8 0.85 0.9 0.95 1 1 1 1 1 1
  line L7 (5.2543, -2.1305) -> (6.7457, -1.8695)
  line L8 (5.1294, -4.8986) -> (4.2311, -6.0172)
  line L9 (-4.7019, -5.4579) -> (-4.6802, -7.2858)
  line L10 (4.6802, -5.4579) -> (4.6802, -7.2739)
  line L11 (-3.6802, -8.2739) -> (3.6802, -8.2739)
  arc A0 (-4.6802, -7.2858) -> (-3.6802, -8.2739) centre (-3.6802, -7.2739) ccw
  arc A1 (3.6802, -8.2739) -> (4.6802, -7.2739) centre (3.6802, -7.2739) ccw
  line L12 (-3.6802, -8.2739) -> (3.6802, -8.2739)
  arc A2 (-2.3308, -22.3896) -> (-3.6802, -8.2739) centre (-54.9016, -20.2929) ccw
  arc A3 (3.6798, -8.2739) -> (2.3308, -22.3896) centre (54.9071, -20.2919) ccw
  line L13 (-5, -22.3896) -> (5, -22.3896)
  line L14 (5, -22.3896) -> (5, -22.6986)
  line L15 (4.059, -23.6396) -> (-4.059, -23.6396)
  line L16 (-5, -22.6986) -> (-5, -22.3896)
  arc A4 (-5, -22.6986) -> (-4.059, -23.6396) centre (-4.059, -22.6986) ccw
  arc A5 (4.059, -23.6396) -> (5, -22.6986) centre (4.059, -22.6986) ccw
  line L17 (-4.059, -23.6396) -> (3.9517, -23.6396)
  line L18 (3.9517, -23.6396) -> (3.9517, -23.6817)
  line L19 (2.7437, -24.8896) -> (-2.8511, -24.8896)
  line L20 (-4.059, -23.6817) -> (-4.059, -23.6396)
  arc A6 (-4.059, -23.6817) -> (-2.8511, -24.8896) centre (-2.8511, -23.6817) ccw
  arc A7 (2.7437, -24.8896) -> (3.9517, -23.6817) centre (2.7437, -23.6817) ccw
  line L21 (-2.8511, -24.8896) -> (2.7437, -24.8896)
  line L22 (2.7437, -24.8896) -> (2.7437, -25.6896)
  line L23 (2.7437, -25.6896) -> (-2.8511, -25.6896)
  line L24 (-2.8511, -25.6896) -> (-2.8511, -24.8896)
  line L25 (-2.9946, -25.6896) -> (3.15, -25.6896)
  line L26 (3.15, -25.845) -> (3.15, -25.8342)
  line L27 (2.9946, -25.9896) -> (-2.9946, -25.9896)
  line L28 (-3.15, -25.8342) -> (-3.15, -25.845)
  arc A8 (-3.15, -25.8342) -> (-2.9946, -25.9896) centre (-2.9946, -25.8342) ccw
  arc A9 (-2.9946, -25.6896) -> (-3.15, -25.845) centre (-2.9946, -25.845) ccw
  arc A10 (2.9946, -25.9896) -> (3.15, -25.8342) centre (2.9946, -25.8342) ccw
  arc A11 (3.15, -25.845) -> (2.9946, -25.6896) centre (2.9946, -25.845) ccw
  line L29 (2.8511, -25.9988) -> (-2.8511, -25.9804)
  arc A12 (-5.5, -34.0205) -> (-2.8511, -25.9804) centre (-14.8637, -26.4791) ccw
  arc A13 (-5.5, -34.0205) -> (-2.8511, -25.9804) centre (-14.8637, -26.4791) ccw
  arc A14 (2.8511, -25.9804) -> (5.5, -34.0205) centre (14.8637, -26.4791) ccw
  line L30 (-1.75, -34.0205) -> (1.75, -34.0205)
  line L31 (-1.75, -34.0205) -> (1.7499, -34.0205)
  line L32 (1.7499, -34.0205) -> (1.7499, -34.6869)
  line L33 (-1.75, -34.6869) -> (-1.75, -34.0205)
  arc A15 (-1.75, -34.6869) -> (-1.4743, -34.9942) centre (-1.4409, -34.6869) ccw
  arc A16 (1.4406, -34.996) -> (1.7499, -34.6869) centre (1.4408, -34.6869) ccw
  line L34 (-1.4743, -34.9942) -> (1.4406, -34.996)
  line L35 (0, 0) -> (0, -37)
  line L36 (-0.3, -34.9951) -> (0.3, -34.9951)
  line L37 (-0.3, -34.9951) -> (-0.3, -37.2951)
  line L38 (-0.3, -37.2951) -> (-1.1, -37.2951)
  line L39 (-1.1, -37.2951) -> (-1.1, -37.8951)
  line L40 (-1.1, -37.8951) -> (-0.3, -37.8951)
  line L41 (-0.3, -37.8951) -> (-0.3, -38.7951)
  line L42 (-0.3, -38.7951) -> (0, -38.7951)
  line L43 (0.3, -34.9951) -> (0.3, -37.2951)
  line L44 (0.3, -37.2951) -> (1.1, -37.2951)
  line L45 (1.1, -37.2951) -> (1.1, -37.8951)
  line L46 (1.1, -37.8951) -> (0.3, -37.8951)
  line L47 (0.3, -37.8951) -> (0.3, -38.7951)
  line L48 (0.3, -38.7951) -> (0, -38.7951)
  circle A17 centre (-0.0006, -38.4084) radius 0.2409
  line L49 (0, -38.7951) -> (0, -38.6493)
  point P0 (0, -34.0205)
  point P1 (0, -8.7015)
  point P2 (0, -2)
  point P3 (-7.605, -2.3307)
  point P4 (-8.0306, -3.2451)
  point P5 (-6.9575, -4.0005)
  point P6 (7.605, -2.3307)
  point P7 (8.0306, -3.2451)
  point P8 (6.9575, -4.0005)
  point P9 (0, -22.3896)
  point P10 (0, -8.2739)
  point P11 (-5, -23.6396)
  point P12 (-4.059, -24.8896)
  point P13 (0, -25.6896)
  point P14 (-3.15, -25.9896)
  point P15 (0, -25.9896)
  point P16 (0, -34.0205)
  point P17 (-1.75, -34.7205)
  point P18 (0, -34.9951)
  dimension "d127" = 16
  dimension "d128" = 37
  dimension "d131" = 1
  dimension "d132" = 1.25
  dimension "d133" = 0.941
  dimension "d134" = 1.25
  dimension "d135" = 1.2079
  dimension "d136" = 0.8
  dimension "d139" = 0.1554
  dimension "d140" = 11
  dimension "d141" = 5.7022
  dimension "d142" = 3.5
  dimension "d143" = 0.7
  dimension "d144" = 0.3091
  dimension "d162" = 0.6
  dimension "d163" = 2.3
  dimension "d164" = 0.8
  dimension "d165" = 0.6
  dimension "d166" = 0.8
  dimension "d167" = 0.9
  constraint midpoint L0 L1.start
  constraint coincident L1.start L35.start
  constraint horizontal L0
  constraint perpendicular L0 L1
  constraint midpoint L2 P16
  constraint coincident L1 P16
  constraint perpendicular L1 L2
  constraint coincident L1 P1
  constraint midpoint L3 P2
  constraint coincident L1 P2
  constraint perpendicular L1 L3
  constraint midpoint L3.start L4
  constraint perpendicular L10 L11
  constraint tangent L9 A0
  constraint tangent L11 A0
  constraint tangent L10 A1
  constraint tangent L11 A1
  constraint equal A0 A1
  constraint coincident L1 P9
  constraint midpoint L12 P10
  constraint coincident L11 P10
  constraint horizontal L13
  constraint vertical L14
  constraint horizontal L15
  constraint vertical L16
  constraint coincident P11 L15
  constraint coincident P11 L16
  constraint tangent L15 A4
  constraint tangent L16 A4
  constraint tangent L14 A5
  constraint tangent L15 A5
  constraint equal A4 A5
  constraint horizontal L17
  constraint vertical L18
  constraint horizontal L19
  constraint vertical L20
  constraint coincident P12 L19
  constraint coincident P12 L20
  constraint tangent L19 A6
  constraint tangent L20 A6
  constraint tangent L18 A7
  constraint tangent L19 A7
  constraint equal A6 A7
  constraint horizontal L21
  constraint vertical L22
  constraint horizontal L23
  constraint vertical L24
  constraint coincident L1 P13
  constraint coincident L23 P13
  constraint perpendicular L1 L25
  constraint vertical L26
  constraint horizontal L27
  constraint vertical L28
  constraint coincident P14 L27
  constraint coincident P14 L28
  constraint tangent L27 A8
  constraint tangent L28 A8
  constraint coincident L25 P13
  constraint tangent L25 A9
  constraint tangent L28 A9
  constraint equal A8 A9
  constraint tangent L26 A10
  constraint tangent L27 A10
  constraint equal A8 A10
  constraint tangent L26 A11
  constraint equal A8 A11
  constraint midpoint L29 P15
  constraint coincident L27 P15
  constraint symmetric L1 L2.start L2.end
  constraint symmetric L1 L29.end A14.start
  constraint symmetric L1 A13 A14
  constraint midpoint L30 P16
  constraint coincident P16 P0
  constraint perpendicular L1 L30
  constraint horizontal L31
  constraint vertical L32
  constraint vertical L33
  constraint coincident P17 L33
  constraint tangent L33 A15
  constraint tangent L32 A16
  constraint equal A15 A16
  constraint tangent A16 L34
  constraint symmetric L35.start L1 origin
  constraint symmetric L35.end L1 L1.end
  constraint midpoint L36 P18
  constraint coincident L35 P18
  constraint coincident L34 P18
  constraint perpendicular L35 L36
  constraint perpendicular L36 L37
  constraint perpendicular L37 L38
  constraint perpendicular L38 L39
  constraint perpendicular L39 L40
  constraint perpendicular L40 L41
  constraint perpendicular L41 L42
  constraint symmetric L35 L36.start L36.end
  constraint symmetric L35 L37.end L43.end
  constraint symmetric L35 L38.end L44.end
  constraint symmetric L35 L39.end L45.end
  constraint symmetric L35 L40.end L46.end
  constraint symmetric L35 L41.end L47.end
  constraint symmetric L35 L42.end L48.end
  constraint coincident A17 L49.end
  constraint perpendicular L42 L49
  measures "d127" distance of L0.start L0.end
  measures "d128" distance of L1.start L1.end
  measures "d131" radius of A0
  measures "d132" distance of L13.start P11
  measures "d133" radius of A4
  measures "d134" distance of L15.end P12
  measures "d135" radius of A6
  measures "d136" distance of L19.end L23.end
  measures "d139" radius of A8
  measures "d140" distance of L2.start L2.end
  measures "d141" distance of L29.start L29.end
  measures "d142" distance of L30.start L30.end
  measures "d143" distance of L30.start P17
  measures "d144" radius of A15
  measures "d162" distance of L36.start L36.end
  measures "d163" distance of L36.start L37.end
  measures "d164" distance of L37.end L38.end
  measures "d165" distance of L38.end L39.end
  measures "d166" distance of L39.end L40.end
  measures "d167" distance of L40.end L41.end
revolve "Revolve8" add sketch "King" angle 360 about axis through (0, 0, 1.75) along (0, 0, 1) contours L0 L1 L3 S1 L35 | L1 L3 S3 L10 L11 A1 L12 L35 | L1 L11 L12 A3 L13 L35 | L1 L13 L14 L15 A5 L17 L35 | L1 L15 L17 L18 L19 A7 L21 L35 | L1 L19 L21 L22 L23 L25 L35 | L1 L23 L25 L27 A10 A11 L35 | L1 L2 L29 A14 L30 L31 L35 | L1 L2 L30 L31 L32 A16 L34 L35 L36 makes body 1
extrude "Extrude9" add sketch "King" along normal mid plane 0.646 separate body contours L34 L36 L37 L38 L39 L40 L41 L42 L43 L44 L45 L46 L47 L48 | A17 makes body 2
fillet "Fillet10" radius 0.139 4 edges at (0.3, 0, 37.8951) (0.3, 0, 37.2951) (-0.3, 0, 37.2951) (-0.3, 0, 37.8951) on bodies 2
fillet "Fillet11" radius 0.068 6 edges at (-0.3, 0, 38.7951) (0.3, 0, 38.7951) (1.1, 0, 37.8951) (-1.1, 0, 37.8951) (-1.1, 0, 37.2951) (1.1, 0, 37.2951) on bodies 2
chamfer "Chamfer3" distance 0.057 angle 45 42 edges at (0.3, -0.323, 36.0757) (0.3407, -0.323, 37.2544) (0.7355, -0.323, 37.2951) (1.0801, -0.323, 37.315) (1.1, -0.323, 37.5951) (1.0801, -0.323, 37.8752) (0.7355, -0.323, 37.8951) (0.3407, -0.323, 37.9358) (0.3, -0.323, 38.3806) (0.2801, -0.323, 38.7752) (0, -0.323, 38.7951) (-0.2801, -0.323, 38.7752) (-0.3, -0.323, 38.3806) (-0.3407, -0.323, 37.9358) (-0.7355, -0.323, 37.8951) (-1.0801, -0.323, 37.8752) (-1.1, -0.323, 37.5951) (-1.0801, -0.323, 37.315) (-0.7355, -0.323, 37.2951) (-0.3407, -0.323, 37.2544) (-0.3, -0.323, 36.0756) (0.3, 0.323, 36.0757) (-0.3, 0.323, 36.0756) (-0.3407, 0.323, 37.2544) (-0.7355, 0.323, 37.2951) (-1.0801, 0.323, 37.315) (-1.1, 0.323, 37.5951) (-1.0801, 0.323, 37.8752) (-0.7355, 0.323, 37.8951) (-0.3407, 0.323, 37.9358) (-0.3, 0.323, 38.3806) (-0.2801, 0.323, 38.7752) (0, 0.323, 38.7951) (0.2801, 0.323, 38.7752) (0.3, 0.323, 38.3806) (0.3407, 0.323, 37.9358) (0.7355, 0.323, 37.8951) (1.0801, 0.323, 37.8752) (1.1, 0.323, 37.5951) (1.0801, 0.323, 37.315) (0.7355, 0.323, 37.2951) (0.3407, 0.323, 37.2544) tangent chain off on bodies 2
fillet "Fillet12" radius 0.437 1 edges at (-5.1278, -1.9889, 34.0205) on bodies 1
move_body "Move17" bodies 2 1 to x (1, 0, 0) y (0, 1, 0) z (0, 0, 1) at (-20.1423, 0, 0)
move_body "Move19" bodies 2 1 to x (1, 0, 0) y (0, 1, 0) z (0, 0, 1) at (2.9151, 0, 0)
move_body "Align1" bodies 2 to x (1, 0, 0) y (0, 1, 0) z (0, 0, 1) at (17.2272, 0, 0)
move_body "Align2" bodies 1 to x (1, 0, 0) y (0, 1, 0) z (0, 0, 1) at (17.2272, 0, -12.0197)
move_body "Move20" bodies 1 to x (1, 0, 0) y (0, 1, 0) z (0, 0, 1) at (0, 0, 11.997)
